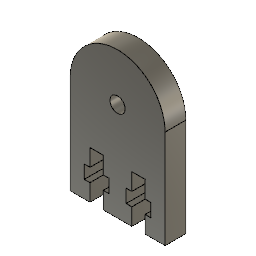
rotor_stand v6 (Autodesk Fusion 360 design; units mm, degrees)
Autodesk Fusion 360 part; units mm, degrees
sketch "Sketch1" plane through (0, 0, 0) normal (0, 1, 0) x (1, 0, 0)
  circle A0 centre (0, 0) radius 4
  circle A1 centre (0, 0) radius 25
  line L0 (0, 0) -> (-25, 0)
  line L1 (0, 0) -> (25, 0)
  line L2 (-25, 0) -> (25, 0)
  line L3 (25, 0) -> (25, 51.781)
  line L4 (25, 51.781) -> (-25, 51.781)
  line L5 (-25, 51.781) -> (-25, 0)
  line L6 (-14.5, 51.781) -> (-7.5, 51.781)
  line L7 (-7.5, 51.781) -> (-7.5, 26.781)
  line L8 (-7.5, 26.781) -> (-14.5, 26.781)
  line L9 (-14.5, 26.781) -> (-14.5, 51.781)
  line L10 (-17.5, 35.781) -> (-4.5, 35.781)
  line L11 (-4.5, 35.781) -> (-4.5, 42.781)
  line L12 (-4.5, 42.781) -> (-17.5, 42.781)
  line L13 (-17.5, 42.781) -> (-17.5, 35.781)
  line L14 (-11, 35.781) -> (-11, 26.781)
  line L15 (-17.5, 39.281) -> (-14.5, 39.281)
  line L16 (0, 51.781) -> (0, 83.1045)
  line L17 (7.5, 51.781) -> (7.5, 26.781)
  line L18 (7.5, 26.781) -> (14.5, 26.781)
  line L19 (14.5, 26.781) -> (14.5, 51.781)
  line L20 (17.5, 35.781) -> (4.5, 35.781)
  line L21 (17.5, 42.781) -> (17.5, 35.781)
  line L22 (4.5, 42.781) -> (17.5, 42.781)
  line L23 (4.5, 35.781) -> (4.5, 42.781)
  dimension "d1" = 8
  dimension "d2" = 50
  dimension "d3" = 25
  dimension "d4" = 7
  dimension "d5" = 7
  dimension "d6" = 13
  dimension "d7" = 90
  dimension "d8" = 90
  dimension "d9" = 9
  dimension "d10" = 51.781
  constraint coincident A0.centre A1.centre
  constraint coincident A1 L0.end
  constraint horizontal L0
  constraint coincident A1 L1.end
  constraint parallel L0 L1
  constraint horizontal L2
  constraint vertical L3
  constraint horizontal L4
  constraint vertical L5
  constraint horizontal L6
  constraint vertical L7
  constraint horizontal L8
  constraint vertical L9
  constraint coincident L4 L6.start
  constraint horizontal L10
  constraint vertical L11
  constraint horizontal L12
  constraint vertical L13
  constraint midpoint L10 L14.start
  constraint midpoint L8 L14.end
  constraint midpoint L13 L15.start
  constraint midpoint L9 L15.end
  constraint midpoint L4 L16.start
  constraint perpendicular L4 L16
  constraint symmetric L6.start L16 L19.end
  constraint symmetric L6.end L16 L17.start
  constraint symmetric L7.end L16 L17.end
  constraint symmetric L8.end L16 L18.end
  constraint symmetric L10.start L16 L20.start
  constraint symmetric L10.end L16 L20.end
  constraint symmetric L11.end L16 L22.start
  constraint symmetric L12.end L16 L21.start
  measures "d1" diameter of A0
  measures "d2" diameter of A1
  measures "d3" distance of L6.end L7.end
  measures "d4" distance of L7.end L8.end
  measures "d5" distance of L10.start L12.end
  measures "d6" distance of L11 L13
  measures "d7" angle of L8 L14
  measures "d8" angle of L9 L15
  measures "d9" distance of L11 L23
  measures "d10" distance of A0.centre L4
extrude "Extrude1" add sketch "Sketch1" along normal blind 10 contours A0 A1 L0 L1 L2 | A0 A1 L0 L1 L2 | A1 L3 L4 L5 L7 L8 L9 L10 L11 L12 L13 L17 L18 L19 L20 L21 L22 L23
extrude "Extrude2" add 1 faces at (14.2683, 0, -9.6781) along direction (0, -1, 0) blind 1
